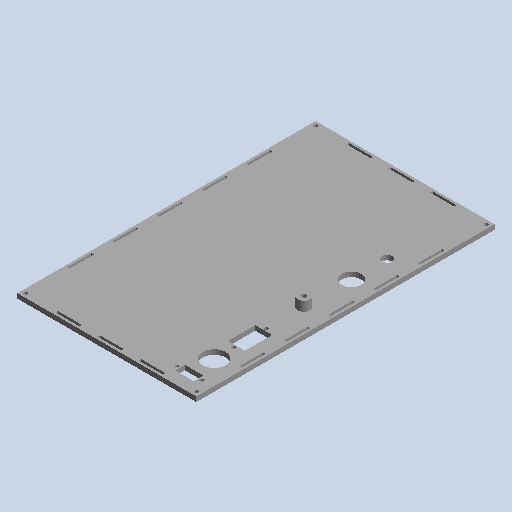
# Autodesk Inventor part: Enclosure_6
Saved by Autodesk Inventor 2026 (Build 300175050, 175E)
## iProperties
Part Number: Enclosure_6
Material: Generic
Document SubType Name: Modeling
Designer: Kartik
Mass: 143.752 g
Surface Area: 792.803 cm^2
Volume: 143.752 cm^3
Density: 1 g/cm^3
Appearance: Default
Author: Kartik
Autodesk Inventor part; units mm, degrees
ref_plane "YZ Plane" through (0, 0, 0) normal (1, 0, 0) x (0, 1, 0)
ref_plane "XZ Plane" through (0, 0, 0) normal (0, 1, 0) x (-1, 0, 0)
ref_plane "XY Plane" through (0, 0, 0) normal (0, 0, 1) x (1, 0, 0)
sketch "Sketch1" plane through (0, 0, 0) normal (0, 1, 0) x (-1, 0, 0)
  line L0 (31.1634, 169.1828) -> (-118.8366, 169.1828)
  line L1 (-118.8366, 169.1828) -> (-118.8366, -80.8172)
  line L2 (-118.8366, -80.8172) -> (31.1634, -80.8172)
  line L3 (31.1634, -80.8172) -> (31.1634, 169.1828)
  point P0 (0, 0)
  dimension "d0" = 250
  dimension "d1" = 150
  constraints: 8 end point, 2 parallel, 1 horizontal, 1 perpendicular
  measures "d0" distance of L2.end L0.start
  measures "d1" distance of L1.end L2.end
extrude "Extrusion1" add sketch "Sketch1" along normal blind 4
fillet "Fillet1" [suppressed]
sketch "Sketch2" plane through (0, 4, 0) normal (0, 1, 0) x (1, 0, 0)
  line L0 (-31.1634, 80.8172) -> (-31.1634, -169.1828) projected
  line L1 (-31.1634, -169.1828) -> (118.8366, -169.1828) projected
  line L2 (118.8366, -169.1828) -> (118.8366, 80.8172) projected
  line L3 (118.8366, 80.8172) -> (-31.1634, 80.8172) projected
  arc A0 (-21.1634, 76.8172) -> (-27.1634, 70.8172) centre (-21.1634, 70.8172) ccw
  arc A1 (114.8366, 70.8172) -> (108.8366, 76.8172) centre (108.8366, 70.8172) ccw
  arc A2 (108.8366, -165.1828) -> (114.8366, -159.1828) centre (108.8366, -159.1828) ccw
  arc A3 (-27.1634, -159.1828) -> (-21.1634, -165.1828) centre (-21.1634, -159.1828) ccw
  line L4 (108.8366, -165.1828) -> (98.8366, -165.1828)
  line L5 (-11.1634, -165.1828) -> (-21.1634, -165.1828)
  line L6 (-27.1634, -159.1828) -> (-27.1634, -149.1828)
  line L7 (-27.1634, 60.8172) -> (-27.1634, 70.8172)
  line L8 (-21.1634, 76.8172) -> (-11.1634, 76.8172)
  line L9 (98.8366, 76.8172) -> (108.8366, 76.8172)
  line L10 (114.8366, 70.8172) -> (114.8366, 60.8172)
  line L11 (114.8366, -149.1828) -> (114.8366, -159.1828)
  line L12 (-11.1634, -169.1828) -> (-11.1634, -165.1828)
  line L13 (-11.1634, 76.8172) -> (-11.1634, 80.8172)
  line L14 (-31.1634, 60.8172) -> (-27.1634, 60.8172)
  line L15 (114.8366, 60.8172) -> (118.8366, 60.8172)
  line L16 (98.8366, -169.1828) -> (98.8366, -165.1828)
  line L17 (98.8366, 76.8172) -> (98.8366, 80.8172)
  line L18 (-31.1634, -149.1828) -> (-27.1634, -149.1828)
  line L19 (114.8366, -149.1828) -> (118.8366, -149.1828)
  point P0 (0, 0)
  point P1 (114.8366, -154.1828)
  dimension "d12" = 4
  dimension "d13" = 20
  dimension "d14" = 4
  constraints: 32 end point, 8 point on circle, 8 point on line, 4 centre point, 4 vertical, 2 horizontal, 2 perpendicular, 1 midpoint
  measures "d12" distance from line of L2 point (114.837, -154.183)
  measures "d13" distance between parallel lines of L2 L16
  measures "d14" distance between parallel lines of L2 L10
extrude "Extrusion2" [suppressed]
sketch "Sketch3" plane through (0, 4, 0) normal (0, 1, 0) x (1, 0, 0)
  line L0 (-29.1634, -129.1828) -> (-27.1634, -129.1828)
  line L1 (-27.1634, -129.1828) -> (-27.1634, -109.1828)
  line L2 (-27.1634, -109.1828) -> (-29.1634, -109.1828)
  line L3 (-29.1634, -109.1828) -> (-29.1634, -129.1828)
  line L4 (-31.1634, 80.8172) -> (-31.1634, -169.1828) projected
  line L5 (-29.1634, -71.6828) -> (-29.1634, -91.6828)
  line L6 (-29.1634, -91.6828) -> (-27.1634, -91.6828)
  line L7 (-27.1634, -91.6828) -> (-27.1634, -71.6828)
  line L8 (-27.1634, -71.6828) -> (-29.1634, -71.6828)
  line L9 (-29.1634, -34.1828) -> (-29.1634, -54.1828)
  line L10 (-29.1634, -54.1828) -> (-27.1634, -54.1828)
  line L11 (-27.1634, -54.1828) -> (-27.1634, -34.1828)
  line L12 (-27.1634, -34.1828) -> (-29.1634, -34.1828)
  line L13 (-29.1634, 3.3172) -> (-29.1634, -16.6828)
  line L14 (-29.1634, -16.6828) -> (-27.1634, -16.6828)
  line L15 (-27.1634, -16.6828) -> (-27.1634, 3.3172)
  line L16 (-27.1634, 3.3172) -> (-29.1634, 3.3172)
  line L17 (-29.1634, 40.8172) -> (-29.1634, 20.8172)
  line L18 (-29.1634, 20.8172) -> (-27.1634, 20.8172)
  line L19 (-27.1634, 20.8172) -> (-27.1634, 40.8172)
  line L20 (-27.1634, 40.8172) -> (-29.1634, 40.8172)
  line L21 (-31.1634, -169.1828) -> (118.8366, -169.1828) projected
  line L22 (114.8366, -129.1828) -> (116.8366, -129.1828)
  line L23 (116.8366, -129.1828) -> (116.8366, -109.1828)
  line L24 (116.8366, -109.1828) -> (114.8366, -109.1828)
  line L25 (114.8366, -109.1828) -> (114.8366, -129.1828)
  line L26 (114.8366, -91.6828) -> (116.8366, -91.6828)
  line L27 (114.8366, -71.6828) -> (114.8366, -91.6828)
  line L28 (116.8366, -71.6828) -> (114.8366, -71.6828)
  line L29 (114.8366, -54.1828) -> (116.8366, -54.1828)
  line L30 (116.8366, -34.1828) -> (114.8366, -34.1828)
  line L31 (114.8366, -34.1828) -> (114.8366, -54.1828)
  line L32 (116.8366, -54.1828) -> (116.8366, -34.1828)
  line L33 (116.8366, -91.6828) -> (116.8366, -71.6828)
  line L34 (114.8366, -16.6828) -> (116.8366, -16.6828)
  line L35 (116.8366, -16.6828) -> (116.8366, 3.3172)
  line L36 (114.8366, 3.3172) -> (114.8366, -16.6828)
  line L37 (116.8366, 3.3172) -> (114.8366, 3.3172)
  line L38 (114.8366, 20.8172) -> (116.8366, 20.8172)
  line L39 (114.8366, 40.8172) -> (114.8366, 20.8172)
  line L40 (116.8366, 40.8172) -> (114.8366, 40.8172)
  line L41 (116.8366, 20.8172) -> (116.8366, 40.8172)
  line L42 (-1.1634, -167.1828) -> (18.8366, -167.1828)
  line L43 (18.8366, -167.1828) -> (18.8366, -165.1828)
  line L44 (18.8366, -165.1828) -> (-1.1634, -165.1828)
  line L45 (-1.1634, -165.1828) -> (-1.1634, -167.1828)
  line L46 (53.8366, -167.1828) -> (53.8366, -165.1828)
  line L47 (53.8366, -165.1828) -> (33.8366, -165.1828)
  line L48 (33.8366, -167.1828) -> (53.8366, -167.1828)
  line L49 (33.8366, -165.1828) -> (33.8366, -167.1828)
  line L50 (88.8366, -167.1828) -> (88.8366, -165.1828)
  line L51 (88.8366, -165.1828) -> (68.8366, -165.1828)
  line L52 (68.8366, -167.1828) -> (88.8366, -167.1828)
  line L53 (68.8366, -165.1828) -> (68.8366, -167.1828)
  line L54 (18.8366, 76.8172) -> (18.8366, 78.8172)
  line L55 (18.8366, 78.8172) -> (-1.1634, 78.8172)
  line L56 (-1.1634, 76.8172) -> (18.8366, 76.8172)
  line L57 (-1.1634, 78.8172) -> (-1.1634, 76.8172)
  line L58 (53.8366, 76.8172) -> (53.8366, 78.8172)
  line L59 (53.8366, 78.8172) -> (33.8366, 78.8172)
  line L60 (33.8366, 76.8172) -> (53.8366, 76.8172)
  line L61 (33.8366, 78.8172) -> (33.8366, 76.8172)
  line L62 (88.8366, 76.8172) -> (88.8366, 78.8172)
  line L63 (88.8366, 78.8172) -> (68.8366, 78.8172)
  line L64 (68.8366, 76.8172) -> (88.8366, 76.8172)
  line L65 (68.8366, 78.8172) -> (68.8366, 76.8172)
  point P0 (0, 0)
  dimension "d15" = 2
  dimension "d16" = 20
  dimension "d17" = 2
  dimension "d21" = 37.5
  dimension "d28" = 144
  dimension "d33" = 20
  dimension "d34" = 2
  dimension "d35" = 2
  dimension "d39" = 35
  dimension "d42" = 244
  constraints: 128 end point, 4 horizontal, 4 parallel, 2 perpendicular, 2 vertical, 112 other
  measures "d15" distance of L2.end L1.end
  measures "d16" distance of L1.end L0.end
  measures "d17" distance between parallel lines of L4 L3
  measures "d21" distance of L2.end L5.start
  measures "d28" distance of L0.start L22.start
  measures "d33" distance of L44.end L43.end
  measures "d34" distance of L43.end L42.end
  measures "d35" distance between parallel lines of L21 L42
  measures "d39" distance of L42.end L46.start
  measures "d42" distance of L42.end L54.start
extrude "Extrusion3" cut sketch "Sketch3" against normal through all
sketch "Sketch4" plane through (0, 4, 0) normal (0, 1, 0) x (1, 0, 0)
  circle A0 centre (98.8366, -134.1828) radius 9.6
  line L0 (118.8366, -169.1828) -> (118.8366, 80.8172) projected
  line L1 (-31.1634, -169.1828) -> (118.8366, -169.1828) projected
  line L2 (91.7366, -92.6828) -> (105.9366, -92.6828)
  line L3 (105.9366, -92.6828) -> (105.9366, -115.6828)
  line L4 (105.9366, -115.6828) -> (91.7366, -115.6828)
  line L5 (91.7366, -115.6828) -> (91.7366, -92.6828)
  circle A1 centre (98.8366, -19.1828) radius 8.1
  line L6 (-31.1634, 80.8172) -> (-31.1634, -169.1828) projected
  circle A2 centre (98.8366, 10.8172) radius 4.1
  line L7 (90.9866, -150.9828) -> (106.6866, -150.9828)
  line L8 (106.6866, -150.9828) -> (106.6866, -159.1828)
  line L9 (106.6866, -159.1828) -> (90.9866, -159.1828)
  line L10 (90.9866, -159.1828) -> (90.9866, -150.9828)
  circle A3 centre (98.8366, -117.6828) radius 1.5
  circle A4 centre (98.8366, -90.6828) radius 1.5
  circle A5 centre (109.0866, -155.0828) radius 1.5
  circle A6 centre (88.5866, -155.0828) radius 1.5
  point P0 (0, 0)
  point P1 (105.9366, -104.1828)
  point P2 (98.8366, -115.6828)
  point P3 (91.7366, -104.1828)
  point P4 (98.8366, -150.9828)
  dimension "d47" = 19.2
  dimension "d50" = 20
  dimension "d51" = 35
  dimension "d52" = 14.2
  dimension "d53" = 23
  dimension "d54" = 30
  dimension "d56" = 0
  dimension "d57" = 16.2
  dimension "d59" = 130
  dimension "d60" = 150
  dimension "d61" = 8.2
  dimension "d62" = 30
  dimension "d73" = 15.7
  dimension "d74" = 8.2
  dimension "d75" = 0
  dimension "d76" = 10
  dimension "d89" = 3
  dimension "d90" = 3
  dimension "d91" = 27
  dimension "d92" = 13.5
  dimension "d93" = 3
  dimension "d94" = 3
  dimension "d95" = 20.5
  dimension "d96" = 10.25
  constraints: 16 end point, 7 centre point, 4 midpoint, 4 parallel, 2 horizontal, 2 perpendicular
  measures "d47" diameter of A0
  measures "d50" distance from line of L0 A0.centre
  measures "d51" distance from line of L1 A0.centre
  measures "d52" distance of L3.end L4.end
  measures "d53" distance of L2.end L3.end
  measures "d54" vertical distance of point (105.937, -104.183) A0.centre
  measures "d56" horizontal distance of point (98.837, -115.683) A0.centre
  measures "d57" diameter of A1
  measures "d59" distance from line of L6 A1.centre
  measures "d60" distance from line of L1 A1.centre
  measures "d61" diameter of A2
  measures "d62" distance of A2.centre A1.centre
  measures "d73" distance of L8.end L9.end
  measures "d74" distance of L7.end L8.end
  measures "d75" horizontal distance of A0.centre point (98.837, -150.983)
  measures "d76" distance between parallel lines of L1 L9
  measures "d89" diameter of A3
  measures "d90" diameter of A4
  measures "d91" distance of A3.centre A4.centre
  measures "d92" vertical distance of point (91.737, -104.183) A4.centre
  measures "d93" diameter of A5
  measures "d94" diameter of A6
  measures "d95" distance of A6.centre A5.centre
  measures "d96" horizontal distance of point (98.837, -150.983) A6.centre
extrude "Extrusion4" cut sketch "Sketch4" against normal blind 10
sketch "Sketch5" plane through (0, 4, 0) normal (0, 1, 0) x (1, 0, 0)
  circle A0 centre (98.8366, -59.1828) radius 5
  circle A1 centre (98.8366, -19.1828) radius 8.1 projected
  point P0 (0, 0)
  dimension "d63" = 10
  dimension "d77" = 40
  constraints: 1 centre point
  measures "d63" diameter of A0
  measures "d77" distance of A0.centre A1.centre
extrude "Extrusion5" add sketch "Sketch5" along normal blind 8 contours A0
sketch "Sketch6" plane through (98.8366, 12, 59.1828) normal (0, 1, 0) x (1, 0, 0)
  circle A0 centre (0, 0) radius 5 projected
  point P0 (-98.8366, 59.1828)
  constraints: 1 coincident
hole "Hole1" at (98.8366, 12, 59.1828) direction (0, -1, 0) diameter 4 depth 6
sketch "Sketch7" plane through (0, 4, 0) normal (0, 1, 0) x (1, 0, 0)
  circle A0 centre (-27.6634, 77.3172) radius 1.5
  line L0 (118.8366, 80.8172) -> (-31.1634, 80.8172) projected
  line L1 (-31.1634, 80.8172) -> (-31.1634, -169.1828) projected
  point P0 (0, 0)
  dimension "d78" = 3
  dimension "d79" = 3.5
  dimension "d80" = 3.5
  constraints: 1 centre point
  measures "d78" diameter of A0
  measures "d79" distance from line of A0.centre L0
  measures "d80" distance from line of L1 A0.centre
extrude "Extrusion6" cut sketch "Sketch7" against normal blind 10
pattern_linear "Rectangular Pattern1" count 2 spacing 243 along (0, 0, 1) count 2 spacing 143 along (1, 0, 0) of "Extrusion6"
equation "\"d96\" = 0.5 * d95"
body "Solid1"
